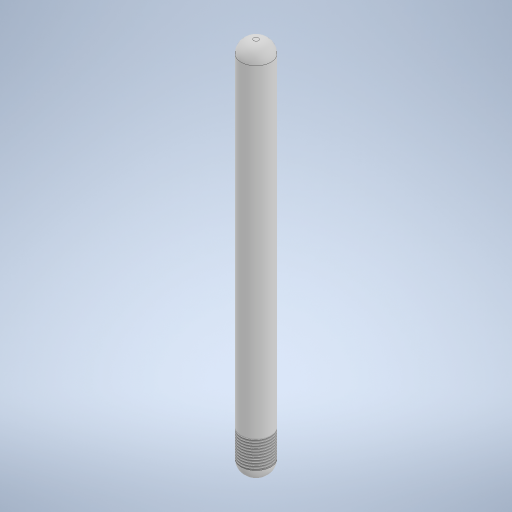
# Autodesk Inventor part: Griff
Saved by Autodesk Inventor 2023.2 (Build 272271030, 271C)
## iProperties
Created: 2023-02-12
Part Number: Griff
Material: Generic
Document SubType Name: Modeling
Designer: Ayush
Density: 1 g/cm^3
Appearance: Default
Author: Ayush
Autodesk Inventor part; units mm, degrees
ref_plane "YZ Plane" through (0, 0, 0) normal (1, 0, 0) x (0, 1, 0)
ref_plane "XZ Plane" through (0, 0, 0) normal (0, 1, 0) x (-1, 0, 0)
ref_plane "XY Plane" through (0, 0, 0) normal (0, 0, 1) x (1, 0, 0)
sketch "Sketch1" plane through (0, 0, 0) normal (0, 1, 0) x (-1, 0, 0)
  circle A0 centre (0, 0) radius 6
  dimension "d0" = 12
  constraints: 1 centre point, 1 coincident
  measures "d0" diameter of A0
extrude "Extrusion1" add sketch "Sketch1" along normal blind 150
fillet "Fillet1" radius 5 1 edges at (6, 150, 0)
fillet "Fillet2" radius 5 1 edges at (6, 0, 0)
thread "Thread1" size "M12x1" class "6g" standard "ANSI Metric M Profile" length 11
body "Solid1"
